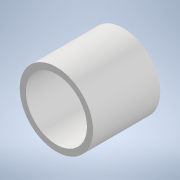
# Autodesk Inventor part: raczka
Saved by Autodesk Inventor 2021 (Build 250183000, 183)
## iProperties
Created: 2021-06-22
Part Number: raczka
Material: Aluminium 6061
Document SubType Name: Modeling
Designer: Wojciech Wołczek
Density: 2.7 g/cm^3
Appearance: Aluminium — płaski
Author: Wojciech Wołczek
Autodesk Inventor part; units mm, degrees
ref_plane "YZ Plane" through (0, 0, 0) normal (1, 0, 0) x (0, 1, 0)
ref_plane "XZ Plane" through (0, 0, 0) normal (0, 1, 0) x (-1, 0, 0)
ref_plane "XY Plane" through (0, 0, 0) normal (0, 0, 1) x (1, 0, 0)
sketch "Szkic1" plane through (0, 0, 0) normal (0, 0, 1) x (1, 0, 0)
  circle A0 centre (0, 0) radius 3 projected
  circle A1 centre (0, 0) radius 6
  point P0 (0, 0)
  dimension "d0" = 12
  constraints: 1 centre point, 1 coincident
  measures "d0" diameter of A1
extrude "Wyciągnięcie proste1" add sketch "Szkic1" against normal blind 1 contours A0 | A1
sketch "Szkic2" plane through (0, 0, 0) normal (0, 0, 1) x (1, 0, 0)
  circle A0 centre (0, 0) radius 6 projected
  circle A1 centre (0, 0) radius 5
  point P0 (0, 0)
  dimension "d3" = 1
  constraints: 1 centre point
  measures "d3" radial gap between concentric circles of A0 A1
extrude "Wyciągnięcie proste2" add sketch "Szkic2" along normal blind 10
full round fillet "Zaokrąglenie1" first side at (4.9353, -0.8021, 6.6667) centre faces at (5.6086, -0.4786, 10) second side at (5.9223, -0.9625, 2.6667)
sketch "Szkic3" plane through (0, 0, 0) normal (0, 1, 0) x (-1, 0, 0)
  line L0 (-6, -1) -> (6, -1) projected
  line L1 (6, 9.5) -> (-6, 9.5) projected
  line L2 (0, 3) -> (25, 3)
  line L3 (25, 3) -> (25, -17)
  line L4 (25, -17) -> (0, -17)
  line L5 (0, -17) -> (0, 3)
  line L6 (0, 3) -> (5.5, 3)
  line L7 (5.5, 3) -> (5.5, -1)
  line L8 (5.5, -1) -> (0, -1)
  line L9 (0, -1) -> (0, 3)
  point P0 (0, 0)
  point P1 (5.5, -1)
  point P2 (0, -1)
  dimension "d6" = 25
  dimension "d7" = 20
  dimension "d8" = 5.5
  dimension "d9" = 4
  constraints: 16 end point, 4 parallel, 2 horizontal, 2 perpendicular, 1 collinear
  measures "d6" distance of L3.end L4.end
  measures "d7" distance of L2.end L3.end
  measures "d8" distance of L7.end L8.end
  measures "d9" distance of L6.end L7.end
extrude "Wyciągnięcie proste3" add sketch "Szkic3" along normal mid plane 2 contours L0 L7 L2 L3 L4 L5
fillet "Zaokrąglenie2" radius 5 1 edges at (-6, 0, 3)
full round fillet "Zaokrąglenie3" first side at (-20.3316, -0.1112, 3) centre faces at (-25, 0.3333, -10.3333) second side at (-8.3333, -0.3333, -17)
pattern_circular "Szyk kołowy1" count 2 over 360 about axis through (0, 0, 0) along (0, 0, 1) of "Wyciągnięcie proste3", "Zaokrąglenie2", "Zaokrąglenie3"
